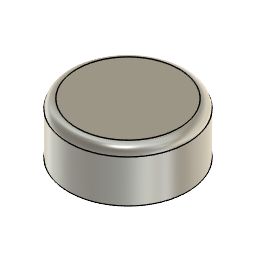
bottle_cap (Autodesk Fusion 360 design; units mm, degrees)
part number: 2025-09-29-07-06-12-361
Autodesk Fusion 360 part; units mm, degrees
sketch "Sketch1" plane through (0, 0, 0) normal (0, 0, 1) x (1, 0, 0)
  circle A0 centre (0, 0) radius 14
  dimension "d1" = 28
  constraint coincident A0.centre origin
  measures "d1" diameter of A0
extrude "Extrude1" add sketch "Sketch1" along normal blind 12
sketch "Sketch4" plane through (0, 0, 0) normal (0, 0, -1) x (1, 0, 0)
  circle A0 centre (0, 0) radius 14
  circle A1 centre (0, 0) radius 12.5
  dimension "d5" = 25
  constraint coincident A0.centre A1.centre
  measures "d5" diameter of A1
hole "Hole1" at (0, 0, 0) direction (0, 0, 1) diameter 25 depth 10 tip angle 180
thread "Thread1" "ISO Metric profile 25.0 M25x1.5 M25x1.5 6H" major diameter 25.208 minor diameter 23.526 pitch 1.5 angle 60 resizes the face on face at (0.6231, 12.4845, 3.3333)
fillet "Fillet1" radius 2 1 edges at (-13.0526, -5.0626, 12)
